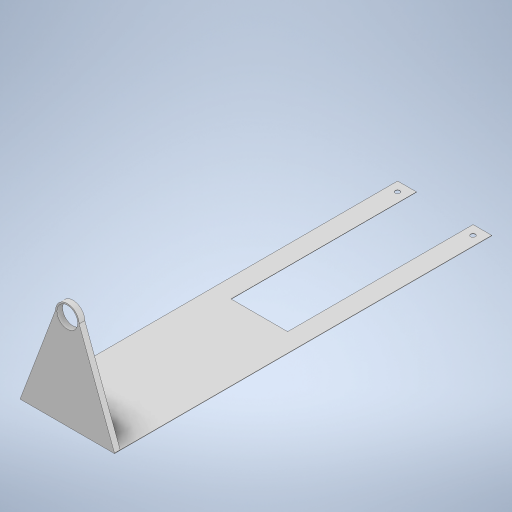
# Autodesk Inventor part: Suporte Central
Saved by Autodesk Inventor 2024 (Build 280153000, 153)
## iProperties
Created: 2024-05-05
Part Number: Suporte Central
Material: Genérico
Document SubType Name: Modeling
Designer: mathe
Density: 1 g/cm^3
Appearance: Padrão
Author: mathe
Autodesk Inventor part; units mm, degrees
ref_plane "YZ Plane" through (0, 0, 0) normal (1, 0, 0) x (0, 1, 0)
ref_plane "XZ Plane" through (0, 0, 0) normal (0, 1, 0) x (-1, 0, 0)
ref_plane "XY Plane" through (0, 0, 0) normal (0, 0, 1) x (1, 0, 0)
sketch "Esboço1" plane through (0, 0, 0) normal (0, 0, 1) x (1, 0, 0)
  line L0 (-21.5807, -22.7321) -> (78.4193, -22.7321)
  line L1 (78.4193, -22.7321) -> (78.4193, -23.0321)
  line L2 (78.4193, -23.0321) -> (-21.5807, -23.0321)
  line L3 (-21.5807, -23.0321) -> (-21.5807, -22.7321)
  circle A0 centre (28.4193, 77.2679) radius 11
  circle A1 centre (28.4193, 77.2679) radius 12.5
  line L4 (-21.5807, -23.0321) -> (17.4193, 77.2679)
  line L5 (15.9193, 77.2679) -> (-21.5807, -22.7321)
  line L6 (39.4193, 77.2679) -> (78.4193, -23.0321)
  line L7 (78.4193, -22.7321) -> (40.9193, 77.2679)
  point P0 (28.4193, -22.7321)
  point P1 (78.3026, -22.7321)
  point P2 (-21.4641, -22.7321)
  dimension "d1" = 100
  dimension "d2" = 0.3
  dimension "d4" = 22
  dimension "d5" = 50
  dimension "d6" = 100
  dimension "d7" = 25
  constraints: 16 end point, 4 point on circle, 2 centre point, 2 parallel, 1 coincident, 1 horizontal, 1 midpoint, 1 perpendicular
  measures "d1" distance of L1.end L2.end
  measures "d2" distance between parallel lines of L2 L0
  measures "d4" diameter of A0
  measures "d5" distance from line of L1 A0.centre
  measures "d6" distance from line of L0 A0.centre
  measures "d7" diameter of A1
extrude "Extrusão1" add sketch "Esboço1" against normal blind 400 contours L0 L6 L2 L4
extrude "Extrusão2" add sketch "Esboço1" against normal blind 6 contours L5 A1 L4 L0 | L4 A1 L6 L0 | A1 L6 A0 L4 | L6 A1 L7 L0 | L4 A0 L6 A1
sketch "Esboço2" plane through (-21.4641, -22.7321, -400) normal (0, 1, 0) x (1, 0, 0)
  line L0 (0, 0) -> (99.7667, 0) projected
  line L1 (20, -196.5848) -> (80, -196.5848)
  line L2 (80, -196.5848) -> (80, 0)
  line L3 (80, 0) -> (20, 0)
  line L4 (20, 0) -> (20, -196.5848)
  line L5 (0, -394) -> (0, 0) projected
  line L6 (99.7667, -394) -> (99.7667, 0) projected
  point P0 (21.4641, -400)
  point P1 (20, 0)
  dimension "d12" = 60
  dimension "d19" = 20
  dimension "d20" = 19.7667
  dimension "d21" = 99.7667
  constraints: 8 end point, 2 parallel, 1 horizontal, 1 perpendicular, 1 point on line
  measures "d12" distance of L3.end L2.end
  measures "d19" distance between parallel lines of L4 L5
  measures "d20" distance between parallel lines of L6 L2
  measures "d21" distance between parallel lines of L6 L5
extrude "Extrusão3" cut sketch "Esboço2" against normal through all
sketch "Esboço3" plane through (-21.4641, -22.7321, -6) normal (0, 1, 0) x (1, 0, 0)
  circle A0 centre (9.8833, 384) radius 2.5
  circle A1 centre (89.8833, 384) radius 2.5
  line L0 (80, 394) -> (99.7667, 394) projected
  line L1 (-0.1167, -6) -> (-0.1167, 394) projected
  line L2 (0, 394) -> (20, 394) projected
  line L3 (99.8833, -6) -> (99.8833, 394) projected
  point P0 (21.4641, -6)
  dimension "d16" = 5
  dimension "d17" = 5
  dimension "d18" = 10
  dimension "d22" = 10
  dimension "d23" = 10
  dimension "d24" = 10
  constraints: 2 centre point
  measures "d16" diameter of A0
  measures "d17" diameter of A1
  measures "d18" distance from line of L0 A1.centre
  measures "d22" distance from line of L1 A0.centre
  measures "d23" distance from line of L2 A0.centre
  measures "d24" distance from line of A1.centre L3
hole "Furo1" at (68.4193, -22.7321, -390) at (-11.5807, -22.7321, -390) direction (0, -1, 0) diameter 5 end through all
